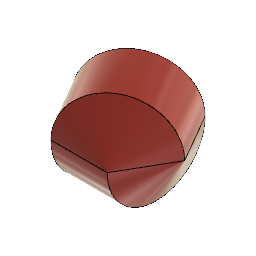
Hexasphericon (Autodesk Fusion 360 design; units mm, degrees)
Autodesk Fusion 360 part; units mm, degrees
sketch "Profile" plane through (0, 0, 0) normal (0, 0, 1) x (1, 0, 0)
  line L0 (50, 0) -> (25, 43.3013)
  line L1 (25, 43.3013) -> (-25, 43.3013)
  line L2 (-25, 43.3013) -> (-50, 0)
  line L3 (-50, 0) -> (-25, -43.3013)
  line L4 (-25, -43.3013) -> (25, -43.3013)
  line L5 (25, -43.3013) -> (50, 0)
  line L6 (-50, 0) -> (50, 0)
  dimension "d1" = 50
revolve "Revolve1" add sketch "Profile" angle 360 about axis through (-50, 0, 0) along (1, 0, 0) contours L0 L1 L2 L6 makes body 1
split "Split1" by plane through (0, 0, 0) normal (0, 0, 1) bodies 1 makes body 2 at (-8.3333, -33.1707, 27.8335)
move_body "Move1" bodies 2 to x (0.5, -0.866025, 0) y (0.866025, 0.5, 0) z (0, 0, 1) at (0, 0, 0)
sketch "Holes" plane through (0, 0, 0) normal (0, 0, 1) x (1, 0, 0)
  circle A0 centre (0, 0) radius 5
  circle A1 centre (0, 0) radius 20 construction
  circle A2 centre (20, 0) radius 2.6
  circle A3 centre (10, 17.3205) radius 2.6
  circle A4 centre (-10, 17.3205) radius 2.6
  circle A5 centre (-20, 0) radius 2.6
  circle A6 centre (-10, -17.3205) radius 2.6
  circle A7 centre (10, -17.3205) radius 2.6
  dimension "d4" = 10
  dimension "d5" = 40
  dimension "d6" = 5.2
  dimension "d8" = 360
  measures "d4" diameter of A0
  measures "d5" diameter of A1
  measures "d6" diameter of A2
extrude "Extrude1" cut sketch "Holes" along normal mid plane 30 contours A0 bodies 1 2
extrude "Extrude2" cut sketch "Holes" along normal mid plane 12 contours A2 | A3 | A4 | A5 | A6 | A7 bodies 1 2
chamfer "Chamfer1" distance 2.5 angle 45 6 edges at (17.5759, -0.9402, 6) (7.5759, -18.2607, 6) (-12.4241, -18.2607, 6) (-22.4241, -0.9402, 6) (-12.4241, 16.3803, 6) (7.5759, 16.3803, 6) on bodies 2
named bodies: "Bottom", "Top"
